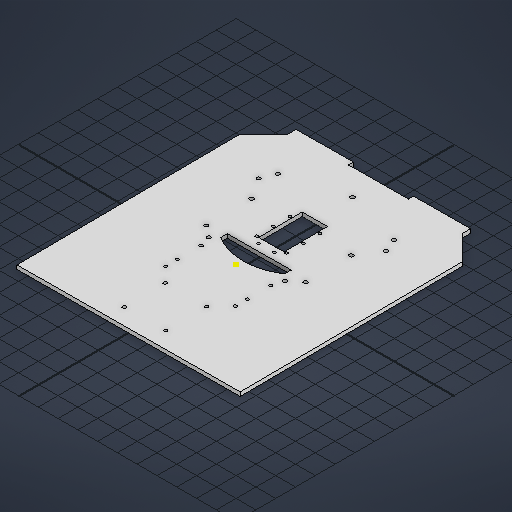
# Autodesk Inventor part: 000.010.001 - Секция центральная
Saved by Autodesk Inventor 2025 (Build 290162000, 162)
## iProperties
Created: 2024-08-22
Part Number: 000.010.001 - Секция центральная
Material: Типовые
Document SubType Name: Modeling
Designer: IvanPetrov
Density: 1 g/cm^3
Appearance: По умолчанию
Author: IvanPetrov
Autodesk Inventor part; units mm, degrees
ref_plane "YZ Plane" through (0, 0, 0) normal (1, 0, 0) x (0, 1, 0)
ref_plane "XZ Plane" through (0, 0, 0) normal (0, 1, 0) x (-1, 0, 0)
ref_plane "XY Plane" through (0, 0, 0) normal (0, 0, 1) x (1, 0, 0)
sketch "Эскиз1" plane through (0, 0, 0) normal (0, 1, 0) x (-1, 0, 0)
  line L0 (-109.5, 112) -> (109.5, 112)
  line L1 (109.5, 112) -> (109.5, -112)
  line L2 (109.5, -112) -> (-109.5, -112)
  line L3 (-109.5, -112) -> (-109.5, 112)
  line L4 (-109.5, 112) -> (109.5, -112) construction
  line L5 (109.5, 112) -> (-109.5, -112) construction
  point P0 (0, 0)
  dimension "d0" = 219
  dimension "d1" = 224
  constraints: 12 end point, 2 midpoint, 2 parallel, 1 horizontal, 1 perpendicular
  measures "d0" distance of L1.end L2.end
  measures "d1" distance of L0.end L1.end
extrude "Выдавливание1" add sketch "Эскиз1" along normal blind 4
sketch "Эскиз2" plane through (0, 0, 0) normal (0, -1, 0) x (1, 0, 0)
  line L0 (-141.5, -87.5) -> (-117, -112)
  line L1 (-150, -87.5) -> (-150, 87.5)
  line L2 (-141.5, 87.5) -> (-117, 112)
  line L3 (-109.5, -112) -> (-109.5, 112) projected
  line L4 (-117, 112) -> (-109.5, 112)
  line L5 (-117, -112) -> (-109.5, -112)
  line L6 (-141.5, -87.5) -> (-150, -87.5)
  line L7 (-141.5, 87.5) -> (-150, 87.5)
  point P0 (0, 0)
  point P1 (-150, -79)
  point P2 (-150, 79)
  constraints: 14 end point, 2 point on line, 1 horizontal, 1 perpendicular
extrude "Выдавливание2" add sketch "Эскиз2" against normal blind 4
sketch "Эскиз3" plane through (0, 0, 0) normal (0, -1, 0) x (1, 0, 0)
  line L0 (-23.5, -32) -> (-23.5, -15) projected
  line L1 (-23.5, 15) -> (-23.5, 32) projected
  arc A0 (-7.5, -0.0017) -> (-125.5, 0.0001) centre (-66.5, -0.0008) ccw projected
  arc A1 (-125.5, -0.0001) -> (-7.5, 0.0017) centre (-66.5, 0.0008) ccw projected
  line L2 (-23.5, 32) -> (-16.9324, 32)
  line L3 (-23.5, 15) -> (-23.5, -15)
  line L4 (-23.5, -32) -> (-16.9324, -32)
  point P0 (0, 0)
  point P1 (-7.5, 0)
  constraints: 6 end point, 2 horizontal, 2 point on circle, 1 perpendicular
extrude "Выдавливание3" cut sketch "Эскиз3" against normal blind 4 contours L0 L3 L1 L2 A0 A1 L4 picked at (-18.1667, 0.0002)
sketch "Эскиз4" plane through (0, 0, 0) normal (0, -1, 0) x (1, 0, 0)
  point P0 (0, 0)
sketch "Эскиз5" plane through (0, 0, 0) normal (0, -1, 0) x (1, 0, 0)
  line L0 (-145, -30) -> (-155, -30)
  line L1 (-155, -30) -> (-155, 30)
  line L2 (-155, 30) -> (-145, 30)
  line L3 (-145, 30) -> (-145, -30)
  line L4 (-150, 87.5) -> (-150, -87.5) projected
  line L5 (-145, -30) -> (-155, 30) construction
  line L6 (-155, -30) -> (-145, 30) construction
  point P0 (0, 0)
  point P1 (-150, 0)
  dimension "d11" = 10
  dimension "d12" = 60
  constraints: 12 end point, 3 midpoint, 2 parallel, 1 horizontal, 1 perpendicular
  measures "d11" distance of L1.end L2.end
  measures "d12" distance of L0.end L1.end
extrude "Выдавливание4" cut sketch "Эскиз5" against normal blind 10
sketch "Эскиз6" plane through (0, 0, 0) normal (0, -1, 0) x (1, 0, 0)
  circle A0 centre (-66.5, 50) radius 2 projected
  circle A1 centre (-118.5438, 0) radius 2 projected
  circle A2 centre (-66.5, -50) radius 2 projected
  point P0 (0, 0)
extrude "Выдавливание5" cut sketch "Эскиз6" against normal through all
sketch "Эскиз7" plane through (0, 0, 0) normal (0, -1, 0) x (1, 0, 0)
  circle A0 centre (-101.6569, 58.3431) radius 1.85 projected
  circle A1 centre (-88, 64) radius 1.85 projected
  circle A2 centre (-20.1068, 49.8759) radius 1.85 projected
  circle A3 centre (-10.9047, 38.3073) radius 1.85 projected
  circle A4 centre (-10.9047, -38.3073) radius 1.85 projected
  circle A5 centre (-20.1068, -49.8759) radius 1.85 projected
  circle A6 centre (-88, -64) radius 1.85 projected
  circle A7 centre (-101.6569, -58.3431) radius 1.85 projected
  point P0 (0, 0)
extrude "Выдавливание6" cut sketch "Эскиз7" against normal through all
sketch "Эскиз8" plane through (0, 0, 0) normal (0, -1, 0) x (1, 0, 0)
  circle A0 centre (0.25, 35) radius 1.5 projected
  circle A1 centre (24.25, 35) radius 1.5 projected
  circle A2 centre (36.25, 35) radius 1.5 projected
  circle A3 centre (36.25, -35) radius 1.5 projected
  circle A4 centre (24.25, -35) radius 1.5 projected
  circle A5 centre (0.25, -35) radius 1.5 projected
  point P0 (0, 0)
extrude "Выдавливание7" cut sketch "Эскиз8" against normal through all
sketch "Эскиз9" plane through (0, 0, 0) normal (0, -1, 0) x (1, 0, 0)
  circle A0 centre (51.1403, 20.8597) radius 1.6 projected
  circle A1 centre (51.1403, -20.8597) radius 1.6 projected
  circle A2 centre (92.8597, 20.8597) radius 1.6 projected
  circle A3 centre (92.8597, -20.8597) radius 1.6 projected
  point P0 (0, 0)
extrude "Выдавливание8" cut sketch "Эскиз9" against normal through all
sketch "Эскиз10" plane through (0, 4, 0) normal (0, 1, 0) x (1, 0, 0)
  circle A0 centre (-30.7, 7.6983) radius 1.35 projected
  circle A1 centre (-30.7, -8.0755) radius 1.35 projected
  circle A2 centre (-70.2, -15) radius 1.35 projected
  circle A3 centre (-70.2, 15) radius 1.35 projected
  circle A4 centre (-53.2, 15) radius 1.35 projected
  circle A5 centre (-53.2, 15) radius 1.35 projected
  circle A6 centre (-53.2, -15) radius 1.35 projected
  circle A7 centre (-36.2, 15) radius 1.35 projected
  circle A8 centre (-36.2, -15) radius 1.35 projected
  line L0 (-75.7, 5.4554) -> (-75.9, 5.4554) projected
  line L1 (-75.9, 5.4554) -> (-75.9, 1.4554) projected
  line L2 (-75.9, 1.4554) -> (-75.7, 1.4554) projected
  line L3 (-75.7, 1.4554) -> (-75.7, -0.4822) projected
  line L4 (-75.7, -0.4822) -> (-75.9, -0.4822) projected
  line L5 (-75.9, -0.4822) -> (-75.9, -4.4822) projected
  line L6 (-75.9, -4.4822) -> (-75.7, -4.4822) projected
  arc A9 (-72.1929, -7.9893) -> (-75.7, -4.4822) centre (-75.7, -7.9893) ccw projected
  line L7 (-72.1929, -7.9893) -> (-72.1929, -11.4929) projected
  line L8 (-72.1929, -11.4929) -> (-39.1923, -11.4929) projected
  line L9 (-39.1923, -11.4929) -> (-39.19, -7.9887) projected
  arc A10 (-37.2, -5.1715) -> (-39.19, -7.9887) centre (-36.2, -7.9893) ccw projected
  line L10 (-37.2, -5.1715) -> (-37.2, 6.1929) projected
  arc A11 (-39.19, 9.0107) -> (-37.2, 6.1929) centre (-36.2, 9.0107) ccw projected
  line L11 (-39.19, 9.0107) -> (-39.1921, 11.4929) projected
  line L12 (-39.1921, 11.4929) -> (-72.179, 11.4929) projected
  line L13 (-72.179, 11.4929) -> (-72.1448, 9.0182) projected
  arc A12 (-75.7, 5.4554) -> (-72.1448, 9.0182) centre (-75.7, 9.0107) ccw projected
  line L14 (-58, -2) -> (-55.8, -2) projected
  line L15 (-58, 2) -> (-58, -2) projected
  line L16 (-55.8, 2) -> (-58, 2) projected
  line L17 (-55.8, -2) -> (-55.8, 2) projected
  circle A13 centre (-66.5, 0) radius 6.5 projected
  line L18 (-37.2, 11.4929) -> (-75.9, 11.4929)
  line L19 (-75.9, 11.4929) -> (-75.9, -11.4929)
  line L20 (-75.9, -11.4929) -> (-37.2, -11.4929)
  line L21 (-37.2, -11.4929) -> (-37.2, 11.4929)
  point P0 (0, 0)
  constraints: 8 end point, 3 point on line, 2 parallel, 1 horizontal, 1 perpendicular
extrude "Выдавливание9" cut sketch "Эскиз10" against normal blind 10 contours A0 | A1 | A2 | A3 | A4 | A6 | A7 | A8 | A12 L13 L12 L11 A11 L10 A10 L9 L8 L7 A9 L6 L5 L4 L3 L2 L1 L0 | L0 L19 L18 L13 A12 | L2 L3 L4 L19 | L18 L21 A11 L11 | L6 A9 L7 L20 L19 | L21 L20 L9 A10 | L15 L16 L17 L14 | A13
offset faces "Размер1" outward -1.25 faces at (-50.1, 1.3333, -11.4929) (-75.9, 1.3333, -3.831) (-37.2, 2.6667, 3.831) (-63, 1.3333, 11.4929)
offset faces "Размер2" outward -3 faces at (-77.15, 2.6667, -4.2476)
